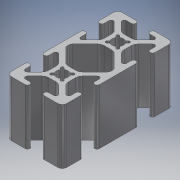
# Autodesk Inventor part: 1020-S
Saved by Autodesk Inventor 2017 SP1 (Build 210196100, 196)
## iProperties
Created: 2016-09-13
Part Number: 1020-S
Material: 6105-T5
Description: 40 S SHORT SINGLE UNIBEARING ASSEMBLY ON 40-4040 X 75mm
Document SubType Name: Modeling
Designer: BRALEF
Density: 1 g/cm^3
Appearance: CLEAR ANODIZED
MATERIAL: 6061-T6
PART PRICE: 44.65
Author: BRALEF
Autodesk Inventor part; units mm, degrees
ref_plane "YZ Plane" through (0, 0, 0) normal (1, 0, 0) x (0, 1, 0)
ref_plane "XZ Plane" through (0, 0, 0) normal (0, 1, 0) x (-1, 0, 0)
ref_plane "XY Plane" through (0, 0, 0) normal (0, 0, 1) x (1, 0, 0)
sketch "Sketch1" plane through (0, 0, 0) normal (0, 1, 0) x (-1, 0, 0)
  arc A0 (9.5718, -14.2658) -> (10.033, -13.1522) centre (8.4582, -13.1522) ccw
  line L0 (10.033, -12.2478) -> (10.033, -13.1522)
  arc A1 (10.033, -12.2478) -> (9.5718, -11.1342) centre (8.4582, -12.2478) ccw
  line L1 (3.8846, -5.4471) -> (9.5718, -11.1342)
  arc A2 (3.8846, -5.4471) -> (1.6396, -4.5172) centre (1.6396, -7.6922) ccw
  line L2 (-1.6396, -4.5172) -> (1.6396, -4.5172)
  arc A3 (-1.6396, -4.5172) -> (-3.8846, -5.4471) centre (-1.6396, -7.6922) ccw
  line L3 (-9.5718, -11.1342) -> (-3.8846, -5.4471)
  arc A4 (-9.5718, -11.1342) -> (-10.033, -12.2478) centre (-8.4582, -12.2478) ccw
  line L4 (-10.033, -13.1522) -> (-10.033, -12.2478)
  arc A5 (-10.033, -13.1522) -> (-9.5718, -14.2658) centre (-8.4582, -13.1522) ccw
  line L5 (-3.8846, -19.9529) -> (-9.5718, -14.2658)
  arc A6 (-3.8846, -19.9529) -> (-1.6396, -20.8828) centre (-1.6396, -17.7078) ccw
  line L6 (1.6396, -20.8828) -> (-1.6396, -20.8828)
  arc A7 (1.6396, -20.8828) -> (3.8846, -19.9529) centre (1.6396, -17.7078) ccw
  line L7 (9.5718, -14.2658) -> (3.8846, -19.9529)
  arc A8 (-1.9692, 2.8605) -> (-2.8605, 1.9692) centre (-2.4696, 2.4696) ccw
  line L8 (-2.2319, 1.3405) -> (-2.8605, 1.9692)
  arc A9 (-2.2319, 1.3405) -> (-2.2319, -1.3405) centre (0, 0) ccw
  line L9 (-2.8605, -1.9692) -> (-2.2319, -1.3405)
  arc A10 (-2.8605, -1.9692) -> (-1.9692, -2.8605) centre (-2.4696, -2.4696) ccw
  line L10 (-1.3405, -2.2319) -> (-1.9692, -2.8605)
  arc A11 (-1.3405, -2.2319) -> (1.3405, -2.2319) centre (0, 0) ccw
  line L11 (1.9692, -2.8605) -> (1.3405, -2.2319)
  arc A12 (1.9692, -2.8605) -> (2.8605, -1.9692) centre (2.4696, -2.4696) ccw
  line L12 (2.2319, -1.3405) -> (2.8605, -1.9692)
  arc A13 (2.2319, -1.3405) -> (2.2319, 1.3405) centre (0, 0) ccw
  line L13 (2.8605, 1.9692) -> (2.2319, 1.3405)
  arc A14 (2.8605, 1.9692) -> (1.9692, 2.8605) centre (2.4696, 2.4696) ccw
  line L14 (1.3405, 2.2319) -> (1.9692, 2.8605)
  arc A15 (1.3405, 2.2319) -> (-1.3405, 2.2319) centre (0, 0) ccw
  line L15 (-1.9692, 2.8605) -> (-1.3405, 2.2319)
  arc A16 (-2.2319, -24.0595) -> (-2.2319, -26.7405) centre (0, -25.4) ccw
  line L16 (-2.8605, -27.3692) -> (-2.2319, -26.7405)
  arc A17 (-2.8605, -27.3692) -> (-1.9692, -28.2605) centre (-2.4696, -27.8696) ccw
  line L17 (-1.3405, -27.6319) -> (-1.9692, -28.2605)
  arc A18 (-1.3405, -27.6319) -> (1.3405, -27.6319) centre (0, -25.4) ccw
  line L18 (1.9692, -28.2605) -> (1.3405, -27.6319)
  arc A19 (1.9692, -28.2605) -> (2.8605, -27.3692) centre (2.4696, -27.8696) ccw
  line L19 (2.2319, -26.7405) -> (2.8605, -27.3692)
  arc A20 (2.2319, -26.7405) -> (2.2319, -24.0595) centre (0, -25.4) ccw
  line L20 (2.8605, -23.4308) -> (2.2319, -24.0595)
  arc A21 (2.8605, -23.4308) -> (1.9692, -22.5395) centre (2.4696, -22.9304) ccw
  line L21 (1.3405, -23.1681) -> (1.9692, -22.5395)
  arc A22 (1.3405, -23.1681) -> (-1.3405, -23.1681) centre (0, -25.4) ccw
  line L22 (-1.9692, -22.5395) -> (-1.3405, -23.1681)
  arc A23 (-1.9692, -22.5395) -> (-2.8605, -23.4308) centre (-2.4696, -22.9304) ccw
  line L23 (-2.2319, -24.0595) -> (-2.8605, -23.4308)
  arc A24 (-10.4902, -4.3561) -> (-12.7, -4.3561) centre (-11.5951, -4.3561) ccw
  line L24 (-10.4902, -4.3561) -> (-10.4902, -6.4749)
  arc A25 (-10.4902, -6.4749) -> (-8.7558, -7.1933) centre (-9.4742, -6.4749) ccw
  line L25 (-8.7558, -7.1933) -> (-5.4471, -3.8846)
  arc A26 (-5.4471, -3.8846) -> (-4.5172, -1.6396) centre (-7.6922, -1.6396) ccw
  line L26 (-4.5172, -1.6396) -> (-4.5172, 1.6396)
  arc A27 (-4.5172, 1.6396) -> (-5.4471, 3.8846) centre (-7.6922, 1.6396) ccw
  line L27 (-5.4471, 3.8846) -> (-8.7558, 7.1933)
  arc A28 (-8.7558, 7.1933) -> (-10.4902, 6.4749) centre (-9.4742, 6.4749) ccw
  line L28 (-10.4902, 6.4749) -> (-10.4902, 4.3561)
  arc A29 (-12.7, 4.3561) -> (-10.4902, 4.3561) centre (-11.5951, 4.3561) ccw
  line L29 (-12.7, 4.3561) -> (-12.7, 10.5918)
  arc A30 (-10.5918, 12.7) -> (-12.7, 10.5918) centre (-10.5918, 10.5918) ccw
  line L30 (-10.5918, 12.7) -> (-4.3561, 12.7)
  arc A31 (-4.3561, 10.4902) -> (-4.3561, 12.7) centre (-4.3561, 11.5951) ccw
  line L31 (-4.3561, 10.4902) -> (-6.4749, 10.4902)
  arc A32 (-6.4749, 10.4902) -> (-7.1933, 8.7558) centre (-6.4749, 9.4742) ccw
  line L32 (-7.1933, 8.7558) -> (-3.8846, 5.4471)
  arc A33 (-3.8846, 5.4471) -> (-1.6396, 4.5172) centre (-1.6396, 7.6922) ccw
  line L33 (-1.6396, 4.5172) -> (1.6396, 4.5172)
  arc A34 (1.6396, 4.5172) -> (3.8846, 5.4471) centre (1.6396, 7.6922) ccw
  line L34 (3.8846, 5.4471) -> (7.1933, 8.7558)
  arc A35 (7.1933, 8.7558) -> (6.4749, 10.4902) centre (6.4749, 9.4742) ccw
  line L35 (6.4749, 10.4902) -> (4.3561, 10.4902)
  arc A36 (4.3561, 12.7) -> (4.3561, 10.4902) centre (4.3561, 11.5951) ccw
  line L36 (4.3561, 12.7) -> (10.5918, 12.7)
  arc A37 (12.7, 10.5918) -> (10.5918, 12.7) centre (10.5918, 10.5918) ccw
  line L37 (12.7, 10.5918) -> (12.7, 4.3561)
  arc A38 (10.4902, 4.3561) -> (12.7, 4.3561) centre (11.5951, 4.3561) ccw
  line L38 (10.4902, 4.3561) -> (10.4902, 6.4749)
  arc A39 (10.4902, 6.4749) -> (8.7558, 7.1933) centre (9.4742, 6.4749) ccw
  line L39 (8.7558, 7.1933) -> (5.4471, 3.8846)
  arc A40 (5.4471, 3.8846) -> (4.5172, 1.6396) centre (7.6922, 1.6396) ccw
  line L40 (4.5172, 1.6396) -> (4.5172, -1.6396)
  arc A41 (4.5172, -1.6396) -> (5.4471, -3.8846) centre (7.6922, -1.6396) ccw
  line L41 (5.4471, -3.8846) -> (8.7558, -7.1933)
  arc A42 (8.7558, -7.1933) -> (10.4902, -6.4749) centre (9.4742, -6.4749) ccw
  line L42 (10.4902, -6.4749) -> (10.4902, -4.3561)
  arc A43 (12.7, -4.3561) -> (10.4902, -4.3561) centre (11.5951, -4.3561) ccw
  line L43 (12.7, -4.3561) -> (12.7, -21.0439)
  arc A44 (10.4902, -21.0439) -> (12.7, -21.0439) centre (11.5951, -21.0439) ccw
  line L44 (10.4902, -21.0439) -> (10.4902, -18.9251)
  arc A45 (10.4902, -18.9251) -> (8.7558, -18.2067) centre (9.4742, -18.9251) ccw
  line L45 (8.7558, -18.2067) -> (5.4471, -21.5154)
  arc A46 (5.4471, -21.5154) -> (4.5172, -23.7604) centre (7.6922, -23.7604) ccw
  line L46 (4.5172, -23.7604) -> (4.5172, -27.0396)
  arc A47 (4.5172, -27.0396) -> (5.4471, -29.2846) centre (7.6922, -27.0396) ccw
  line L47 (5.4471, -29.2846) -> (8.7558, -32.5933)
  arc A48 (8.7558, -32.5933) -> (10.4902, -31.8749) centre (9.4742, -31.8749) ccw
  line L48 (10.4902, -31.8749) -> (10.4902, -29.7561)
  arc A49 (12.7, -29.7561) -> (10.4902, -29.7561) centre (11.5951, -29.7561) ccw
  line L49 (12.7, -29.7561) -> (12.7, -35.9918)
  arc A50 (10.5918, -38.1) -> (12.7, -35.9918) centre (10.5918, -35.9918) ccw
  line L50 (10.5918, -38.1) -> (4.3561, -38.1)
  arc A51 (4.3561, -35.8902) -> (4.3561, -38.1) centre (4.3561, -36.9951) ccw
  line L51 (4.3561, -35.8902) -> (6.4749, -35.8902)
  arc A52 (6.4749, -35.8902) -> (7.1933, -34.1558) centre (6.4749, -34.8742) ccw
  line L52 (7.1933, -34.1558) -> (3.8846, -30.8471)
  arc A53 (3.8846, -30.8471) -> (1.6396, -29.9172) centre (1.6396, -33.0922) ccw
  line L53 (1.6396, -29.9172) -> (-1.6396, -29.9172)
  arc A54 (-1.6396, -29.9172) -> (-3.8846, -30.8471) centre (-1.6396, -33.0922) ccw
  line L54 (-3.8846, -30.8471) -> (-7.1933, -34.1558)
  arc A55 (-7.1933, -34.1558) -> (-6.4749, -35.8902) centre (-6.4749, -34.8742) ccw
  line L55 (-6.4749, -35.8902) -> (-4.3561, -35.8902)
  arc A56 (-4.3561, -38.1) -> (-4.3561, -35.8902) centre (-4.3561, -36.9951) ccw
  line L56 (-4.3561, -38.1) -> (-10.5918, -38.1)
  arc A57 (-12.7, -35.9918) -> (-10.5918, -38.1) centre (-10.5918, -35.9918) ccw
  line L57 (-12.7, -35.9918) -> (-12.7, -29.7561)
  arc A58 (-10.4902, -29.7561) -> (-12.7, -29.7561) centre (-11.5951, -29.7561) ccw
  line L58 (-10.4902, -29.7561) -> (-10.4902, -31.8749)
  arc A59 (-10.4902, -31.8749) -> (-8.7558, -32.5933) centre (-9.4742, -31.8749) ccw
  line L59 (-8.7558, -32.5933) -> (-5.4471, -29.2846)
  arc A60 (-5.4471, -29.2846) -> (-4.5172, -27.0396) centre (-7.6922, -27.0396) ccw
  line L60 (-4.5172, -27.0396) -> (-4.5172, -23.7604)
  arc A61 (-4.5172, -23.7604) -> (-5.4471, -21.5154) centre (-7.6922, -23.7604) ccw
  line L61 (-5.4471, -21.5154) -> (-8.7558, -18.2067)
  arc A62 (-8.7558, -18.2067) -> (-10.4902, -18.9251) centre (-9.4742, -18.9251) ccw
  line L62 (-10.4902, -18.9251) -> (-10.4902, -21.0439)
  arc A63 (-12.7, -21.0439) -> (-10.4902, -21.0439) centre (-11.5951, -21.0439) ccw
  line L63 (-12.7, -21.0439) -> (-12.7, -4.3561)
  point P0 (0, 0)
  dimension "d277" = 1.5748
  dimension "d278" = 3.175
  dimension "d322" = 2.667
  dimension "d323" = 8.1828
  dimension "d324" = 17.2172
  dimension "d325" = 22.733
  dimension "d328" = 8.1828
  dimension "d329" = 17.2172
  dimension "d330" = 33.5828
  dimension "d331" = 42.6172
  dimension "d333" = 15.7509
  dimension "d345" = 20.1702
  dimension "d447" = 2.2096
  dimension "d506" = 1.016
  dimension "d523" = 17.9605
  dimension "d532" = 17.9605
  dimension "d541" = 2.2096
  constraints: 144 tangent, 128 end point, 128 point on circle, 64 centre point, 44 equal radius, 36 parallel, 1 horizontal, 1 perpendicular, 1 vertical
  measures "d277" radius of A1
  measures "d278" radius of A40
  measures "d322" distance between parallel lines of L43 L0
  measures "d323" distance between parallel lines of L43 L46
  measures "d324" distance between parallel lines of L43 L60
  measures "d325" distance between parallel lines of L43 L4
  measures "d328" distance between parallel lines of L36 L33
  measures "d329" distance between parallel lines of L36 L2
  measures "d330" distance between parallel lines of L36 L6
  measures "d331" distance between parallel lines of L36 L53
  measures "d333" distance between parallel lines of L7 L39
  measures "d345" distance between parallel lines of L41 L52
  measures "d447" distance between parallel lines of L34 L39
  measures "d506" radius of A39
  measures "d523" distance between parallel lines of L45 L39
  measures "d532" distance between parallel lines of L47 L41
  measures "d541" distance between parallel lines of L27 L41
extrude "Extrusion1" add sketch "Sketch1" along normal mid plane 25.4
body "Solid1"
